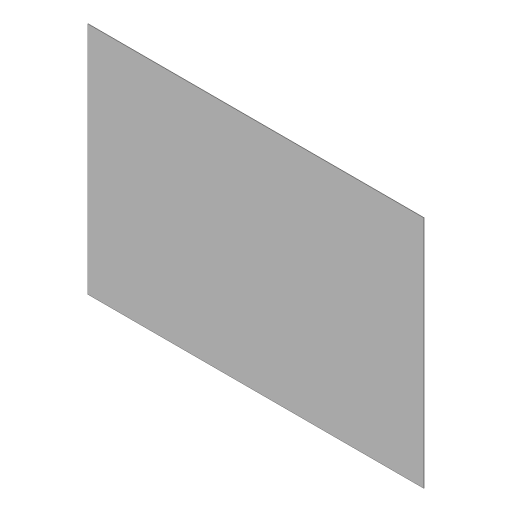
# Autodesk Inventor part: Top_Plate
Saved by Autodesk Inventor 2024.2 (Build 282272000, 272)
## iProperties
Created: 2025-01-06
Part Number: Top_Plate
Material: Generic
Document SubType Name: Sheet Metal
Designer: Kartik
Mass: 219.094 g
Surface Area: 5494.38 cm^2
Volume: 219.094 cm^3
Density: 1 g/cm^3
Sheet Metal Rule: Default_mm
Appearance: Default
Author: Kartik
Autodesk Inventor part; units mm, degrees
ref_plane "YZ Plane" through (0, 0, 0) normal (1, 0, 0) x (0, 1, 0)
ref_plane "XZ Plane" through (0, 0, 0) normal (0, 1, 0) x (-1, 0, 0)
ref_plane "XY Plane" through (0, 0, 0) normal (0, 0, 1) x (1, 0, 0)
sketch "Sketch1" plane through (0, 0, 0) normal (0, 0, 1) x (1, 0, 0)
  line L0 (-313.35, 218.5) -> (313.35, 218.5)
  line L1 (313.35, 218.5) -> (313.35, -218.5)
  line L2 (313.35, -218.5) -> (-313.35, -218.5)
  line L3 (-313.35, -218.5) -> (-313.35, 218.5)
  point P0 (0, 0)
  dimension "d0" = 626.7
  dimension "d1" = 437
  dimension "d2" = 218.5
  dimension "d3" = 313.35
  measures "d0" distance of L0.start L0.end
  measures "d1" distance of L2.end L0.start
  measures "d2" distance from line of L0 point (0, 0)
  measures "d3" distance from line of L3 point (0, 0)
extrude "Plate1" add sketch "Sketch1" along normal blind 0.8
equation "\"d4\" = Thickness"
equation "\"d2\" = 0.5 * d1"
equation "\"d3\" = 0.5 * d0"
equation "\"BendRadius\" = Thickness"
equation "\"BendReliefWidth\" = Thickness"
equation "\"BendReliefDepth\" = 0.5 * Thickness"
equation "\"CornerReliefSize\" = 4 * Thickness"
equation "\"MinimumRemnant\" = 2 * Thickness"
equation "\"TransitionRadius\" = BendRadius"
equation "\"JacobiRadiusSize\" = BendRadius"
equation "\"GapSize\" = Thickness"
equation "\"Thickness\" = 0.8"
body "Solid1"
